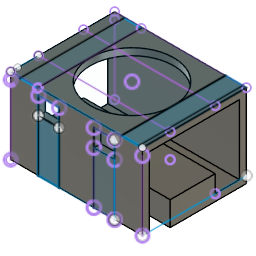
Movement Sensor (Autodesk Fusion 360 design; units mm, degrees)
part number: 2026-08-05-21-35-21-258
Autodesk Fusion 360 part; units mm, degrees
sketch "Sketch1" plane through (0, 0, 0) normal (0, 0, 1) x (1, 0, 0)
  line L0 (0, 0) -> (38, 0)
  line L1 (38, 0) -> (38, 30)
  line L2 (38, 30) -> (0, 30)
  line L3 (0, 30) -> (0, 0)
  line L4 (3, 3) -> (35, 3)
  line L5 (35, 3) -> (35, 27)
  line L6 (35, 27) -> (3, 27)
  line L7 (3, 27) -> (3, 3)
  line L8 (8, 27) -> (32, 27)
  line L9 (32, 27) -> (32, 3)
  line L10 (32, 3) -> (8, 3)
  line L11 (8, 3) -> (8, 27)
  circle A0 centre (20, 15) radius 12
  dimension "d1" = 38
  dimension "d2" = 30
  dimension "d3" = 32
  dimension "d4" = 24
  dimension "d5" = 3
  dimension "d6" = 3
  dimension "d7" = 24
  dimension "d8" = 24
  dimension "d9" = 5
  dimension "d11" = 3
  dimension "d12" = 24
  dimension "d13" = 12
  dimension "d14" = 16.9706
  constraint horizontal L0
  constraint vertical L1
  constraint horizontal L2
  constraint vertical L3
  constraint coincident L0.start L3.end
  constraint horizontal L4
  constraint vertical L5
  constraint horizontal L6
  constraint vertical L7
  constraint horizontal L8
  constraint vertical L9
  constraint horizontal L10
  constraint vertical L11
  measures "d1" distance of L0.start L0.end
  measures "d2" distance of L0.start L2.end
  measures "d3" distance of L4.start L4.end
  measures "d4" distance of L4.start L6.end
  measures "d5" distance of L3 L7
  measures "d6" distance of L2 L6
  measures "d7" distance of L8.start L8.end
  measures "d8" distance of L8.start L10.end
  measures "d9" distance of L7 L11
  measures "d11" distance of L2 L8
  measures "d12" diameter of A0
  measures "d13" distance of L9 A0.centre
  measures "d14" distance of L10.end A0.centre
sketch "Sketch2" plane through (0, 0, 0) normal (0, 1, 0) x (1, 0, 0)
  line L0 (0, 0) -> (38, 0)
  line L1 (38, 0) -> (38, 20)
  line L2 (38, 20) -> (0, 20)
  line L3 (0, 20) -> (0, 0)
  dimension "d15" = 38
  dimension "d16" = 20
  constraint horizontal L0
  constraint vertical L1
  constraint horizontal L2
  constraint vertical L3
  constraint coincident L0.start L3.end
  measures "d15" distance of L0.start L0.end
  measures "d16" distance of L0.start L2.end
sketch "Sketch3" plane through (0, 0, 0) normal (0, 1, 0) x (1, 0, 0)
  line L0 (8, 0) -> (14, 0)
  line L1 (14, 0) -> (14, 20)
  line L2 (14, 20) -> (8, 20)
  line L3 (8, 20) -> (8, 0)
  line L4 (0, 20) -> (0, 0)
  line L5 (24, 0) -> (30, 0)
  line L6 (30, 0) -> (30, 20)
  line L7 (30, 20) -> (24, 20)
  line L8 (24, 20) -> (24, 0)
  dimension "d17" = 6
  dimension "d18" = 20
  dimension "d19" = 8
  dimension "d21" = 6
  dimension "d22" = 20
  dimension "d23" = 10
  constraint horizontal L0
  constraint vertical L1
  constraint horizontal L2
  constraint vertical L3
  constraint horizontal L5
  constraint vertical L6
  constraint horizontal L7
  constraint vertical L8
  measures "d17" distance of L0.start L0.end
  measures "d18" distance of L0.start L2.end
  measures "d19" distance of L3 L4
  measures "d21" distance of L5.start L5.end
  measures "d22" distance of L5.start L7.end
  measures "d23" distance of L1 L8
sketch "Sketch4" plane through (0, 0, 0) normal (0, 1, 0) x (1, 0, 0)
sketch "Sketch5" plane through (0, 0, 0) normal (0, 1, 0) x (1, 0, 0)
sketch "Sketch6" plane through (0, 0, 0) normal (0, 1, 0) x (1, 0, 0)
  line L0 (8, 0) -> (14, 0)
  line L1 (14, 0) -> (14, 5)
  line L2 (14, 5) -> (8, 5)
  line L3 (8, 5) -> (8, 0)
  line L4 (38, 0) -> (38, 20)
  line L5 (14, 20) -> (8, 20)
  line L6 (14, 0) -> (14, 20)
  line L7 (24, 0) -> (30, 0)
  line L8 (30, 0) -> (30, 5)
  line L9 (30, 5) -> (24, 5)
  line L10 (24, 5) -> (24, 0)
  line L11 (38, 20) -> (0, 20)
  line L12 (0, 20) -> (0, 0)
  line L13 (30, 20) -> (24, 20)
  dimension "d24" = 5
  dimension "d25" = 24
  dimension "d26" = 15
  dimension "d27" = 6
  dimension "d28" = 15
  dimension "d29" = 14
  dimension "d30" = 30
  dimension "d31" = 20
  constraint horizontal L0
  constraint vertical L1
  constraint horizontal L2
  constraint vertical L3
  constraint horizontal L7
  constraint vertical L8
  constraint horizontal L9
  constraint vertical L10
  measures "d24" distance of L0.start L2.end
  measures "d25" distance of L1 L4
  measures "d26" distance of L2 L5
  measures "d27" distance of L3 L6
  measures "d28" distance of L9 L11
  measures "d29" distance of L4 L10
  measures "d30" distance of L8 L12
  measures "d31" distance of L7 L13
sketch "Sketch7" plane through (0, 0, 0) normal (1, 0, 0) x (0, 1, 0)
  line L0 (0, 0) -> (30, 0)
  line L1 (30, 0) -> (30, -20)
  line L2 (30, -20) -> (0, -20)
  line L3 (0, -20) -> (0, 0)
  line L4 (0, 0) -> (0, -20)
  line L5 (0, 0) -> (30, 0)
  dimension "d32" = 30
  dimension "d33" = 20
  constraint horizontal L0
  constraint vertical L1
  constraint horizontal L2
  constraint vertical L3
  constraint coincident L0.start L3.end
  measures "d32" distance of L1 L4
  measures "d33" distance of L2 L5
sketch "Sketch8" plane through (0, 0, 0) normal (0, 1, 0) x (1, 0, 0)
  line L0 (0, 20, 30) -> (38, 20, 30)
  line L1 (38, 20, 30) -> (38, 0, 30)
  line L2 (38, 0, 30) -> (0, 0, 30)
  line L3 (0, 0, 30) -> (0, 20, 30)
  dimension "d34" = 38
  dimension "d35" = 20
sketch "Sketch9" plane through (0, 0, 0) normal (1, 0, 0) x (0, 1, 0)
sketch "Sketch10" plane through (0, 30, 0) normal (0, 1, 0) x (-1, 0, 0)
sketch "Sketch11" plane through (0, 0, 0) normal (1, 0, 0) x (0, 1, 0)
  line L0 (0, -20, 38) -> (30, -20, 38)
sketch "Sketch12" plane through (0, 0, 0) normal (0, 0, 1) x (1, 0, 0)
sketch "Sketch13" plane through (0, 0, 0) normal (0, 0, 1) x (1, 0, 0)
sketch "Sketch14" plane through (0, 0, 0) normal (1, 0, 0) x (0, 1, 0)
  line L0 (8, -5) -> (21, -5)
  line L1 (21, -5) -> (21, -20)
  line L2 (21, -20) -> (8, -20)
  line L3 (8, -20) -> (8, -5)
  line L4 (30, -20) -> (30, 0)
  line L5 (0, 0) -> (30, 0)
  line L6 (0, 0) -> (0, -20)
  dimension "d36" = 15
  dimension "d37" = 9
  dimension "d38" = 5
  dimension "d39" = 8
  constraint horizontal L0
  constraint vertical L1
  constraint horizontal L2
  constraint vertical L3
  measures "d36" distance of L0.start L2.end
  measures "d37" distance of L1 L4
  measures "d38" distance of L0 L5
  measures "d39" distance of L3 L6
sketch "Sketch15" plane through (0, 0, 0) normal (1, 0, 0) x (0, 1, 0)
sketch "Sketch16" plane through (0, 0, 0) normal (0, 0, 1) x (1, 0, 0)
sketch "Sketch17" plane through (0, 0, 0) normal (1, 0, 0) x (0, 1, 0)
  line L0 (30, 0) -> (30, -20)
  line L1 (30, -20) -> (30, 0)
sketch "Sketch18" plane through (0, 0, 0) normal (1, 0, 0) x (0, 1, 0)
sketch "Sketch19" plane through (0, 30, 0) normal (0, 1, 0) x (1, 0, 0)
sketch "Sketch20" plane through (0, 0, 0) normal (1, 0, 0) x (0, 1, 0)
extrude "Extrude1" add sketch "Sketch1" along normal blind 2 contours L0 L1 L2 L3 | L4 L6 L7 L11 | L4 L10 L11 A0 | L4 L9 L10 A0 | L6 L8 L11 A0 | L4 L5 L6 L9 | L6 L8 L9 A0 makes body 1
extrude "Extrude2" add sketch "Sketch2" along normal blind 30 bodies 1
extrude "Extrude3" cut sketch "Sketch6" along normal blind 30 bodies 1
sketch "Sketch21" plane through (0, 0, 0) normal (0, -1, 0) x (1, 0, 0)
  line L0 (30, -5) -> (24, -5)
  line L1 (24, -5) -> (24, 0)
  line L2 (24, 0) -> (30, 0)
  line L3 (30, 0) -> (30, -5)
  line L4 (8, 0) -> (14, 0)
  line L5 (14, 0) -> (14, -5)
  line L6 (14, -5) -> (8, -5)
  line L7 (8, -5) -> (8, 0)
  line L8 (38, -20) -> (38, 2)
  line L9 (38, 2) -> (0, 2)
  line L10 (0, 2) -> (0, -20)
  line L11 (0, -20) -> (38, -20)
  line L12 (0, 0) -> (8, 0)
  line L13 (14, 0) -> (24, 0)
  line L14 (30, 0) -> (38, 0)
  constraint coincident L12.start origin
  constraint coincident L4.start L7.end
  constraint coincident L4.end L5.start
  constraint coincident L1.end L2.start
  constraint coincident L2.end L3.start
  constraint coincident L8 L14.end
  constraint perpendicular L8 L14
sketch "Sketch22" plane through (0, 0, 0) normal (0, -1, 0) x (1, 0, 0)
  line L0 (8, -5) -> (8, -20)
  line L1 (8, -20) -> (14, -20)
  line L2 (14, -20) -> (14, -5)
  line L3 (14, -20) -> (24, -20)
  line L4 (24, -20) -> (24, -5)
  line L5 (24, -5) -> (30, -5)
  line L6 (30, -5) -> (30, -20)
  dimension "d48" = 90
  dimension "d49" = 6
  constraint vertical L0
  constraint perpendicular L0 L1
  constraint perpendicular L1 L2
  constraint perpendicular L2 L3
  constraint perpendicular L1 L4
  constraint perpendicular L1 L6
  measures "d48" angle of L4 L5
  measures "d49" distance of L4.end L5.end
sketch "Sketch23" plane through (0, 0, 0) normal (0, -1, 0) x (1, 0, 0)
  line L0 (8, -5) -> (14, -5)
  line L1 (14, -5) -> (14, -20)
  line L2 (14, -20) -> (8, -20)
  line L3 (8, -20) -> (8, -5)
  line L4 (0, -20) -> (0, 0)
  line L5 (8, 0) -> (14, 0)
  line L6 (30, -20) -> (24, -20)
  line L7 (24, 0) -> (30, 0)
  line L8 (30, -5) -> (30, -20)
  line L9 (38, -20) -> (38, 0)
  line L10 (24, -20) -> (24, -5)
  dimension "d50" = 8
  dimension "d51" = 6
  dimension "d52" = 15
  dimension "d53" = 5
  dimension "d54" = 20
  dimension "d55" = 8
  dimension "d56" = 14
  constraint horizontal L0
  constraint vertical L1
  constraint horizontal L2
  constraint vertical L3
  measures "d50" distance of L3 L4
  measures "d51" distance of L1 L3
  measures "d52" distance of L0 L2
  measures "d53" distance of L0 L5
  measures "d54" distance of L6 L7
  measures "d55" distance of L8 L9
  measures "d56" distance of L9 L10
sketch "Sketch24" plane through (0, 0, 0) normal (0, -1, 0) x (1, 0, 0)
  line L0 (30, 0) -> (30, -20)
  constraint vertical L0
sketch "Sketch25" plane through (0, 0, 0) normal (0, 1, 0) x (1, 0, 0)
  line L0 (13.8134, -0.1132) -> (7.8134, -0.1132)
  line L1 (7.8134, -0.1132) -> (7.8134, 19.8868)
  line L2 (7.8134, 19.8868) -> (13.8134, 19.8868)
  line L3 (13.8134, 19.8868) -> (13.8134, -0.1132)
  dimension "d57" = 6
  dimension "d58" = 20
  constraint horizontal L0
  constraint vertical L1
  constraint horizontal L2
  constraint vertical L3
  measures "d57" distance of L0.start L0.end
  measures "d58" distance of L0.start L2.end
extrude "Extrude4" cut sketch "Sketch7" along normal blind 38 bodies 1
extrude "Extrude5" add sketch "Sketch14" along normal blind 38 separate body makes body 2
sketch "Sketch26" plane through (0, 0, 2) normal (0, 0, 1) x (-1, 0, 0)
  circle A0 centre (-20, -15) radius 12
  line L0 (0, -30) -> (0, 0)
  line L1 (0, 0) -> (-38, 0)
  line L2 (-38, 0) -> (-38, -30)
  line L3 (-38, -30) -> (0, -30)
  line L4 (0, -8) -> (-38, -8)
  line L5 (0, 0) -> (-8, 0)
  line L6 (0, -21) -> (-38, -21)
  line L7 (-38, -30) -> (0, -30)
  dimension "d63" = 8
  dimension "d64" = 38
  dimension "d65" = 38
  dimension "d66" = 9
  measures "d63" distance of L4 L5
  measures "d64" distance of L6.start L6.end
  measures "d65" distance of L2.end L0.start
  measures "d66" distance of L6 L7
extrude "Extrude6" add 1 faces at (12.6667, 16.6667, -20) along direction (0, 0, -1) blind 2 on bodies 2 bodies 2
sketch "Sketch27" plane through (0, 0, 2) normal (0, 0, 1) x (-1, 0, 0)
  line L0 (-32, -30.0218) -> (-37, -30.0218)
  line L1 (-37, -30.0218) -> (-37, -0.0218)
  line L2 (-37, -0.0218) -> (-32, -0.0218)
  line L3 (-32, -0.0218) -> (-32, -30.0218)
  line L4 (-3, -29.6627) -> (-8, -29.6627)
  line L5 (-8, -29.6627) -> (-8, 0.3373)
  line L6 (-8, 0.3373) -> (-3, 0.3373)
  line L7 (-3, 0.3373) -> (-3, -29.6627)
  point P0 (-20, -15)
  dimension "d69" = 5
  dimension "d70" = 30
  dimension "d71" = 12
  dimension "d72" = 5
  dimension "d73" = 30
  dimension "d74" = 12
  constraint horizontal L0
  constraint vertical L1
  constraint horizontal L2
  constraint vertical L3
  constraint horizontal L4
  constraint vertical L5
  constraint horizontal L6
  constraint vertical L7
  measures "d69" distance of L0.start L0.end
  measures "d70" distance of L0.start L2.end
  measures "d71" distance of L3 P0
  measures "d72" distance of L4.start L4.end
  measures "d73" distance of L4.start L6.end
  measures "d74" distance of P0 L5
extrude "Extrude7" add sketch "Sketch8" against normal blind 2 contours L0 L1 L2 L3 in plane through (0, 30, 0) normal (0, 1, 0) bodies 1
extrude "Extrude8" add sketch "Sketch21" against normal blind 2 contours L0 L1 L3 L5 L6 L7 L8 L10 L11 L12 L13 L14 bodies 1
sketch "Sketch28" plane through (0, 0, 2) normal (0, 0, 1) x (-1, 0, 0)
  line L0 (-32, -30) -> (-32, 0)
  line L1 (-32, 0) -> (-38, 0)
  line L2 (-38, 0) -> (-38, -30)
  line L3 (-38, -30) -> (-32, -30)
  line L4 (-8, -29.6627) -> (-8, 0.3373)
  line L5 (-38, 0) -> (0, 0)
  line L6 (0, -8) -> (0, -2)
  dimension "d79" = 6
  dimension "d80" = 24
  constraint vertical L0
  constraint perpendicular L0 L1
  constraint perpendicular L1 L2
  constraint horizontal L5
  constraint vertical L6
  measures "d79" distance of L0.end L1.end
  measures "d80" distance of L0 L4
sketch "Sketch29" plane through (0, 0, 0) normal (1, 0, 0) x (0, 1, 0)
  line L0 (30, -20) -> (21, -20)
  line L1 (21, -20) -> (21, -22)
  line L2 (21, -22) -> (30, -22)
  line L3 (30, -22) -> (30, -20)
  line L4 (8, -22) -> (8, -5)
  line L5 (-0.3373, 2) -> (29.6627, 2)
  dimension "d81" = 22
  dimension "d82" = 22
  dimension "d83" = 24
  dimension "d84" = 9
  constraint horizontal L0
  constraint vertical L1
  constraint horizontal L2
  constraint vertical L3
  measures "d81" distance of L2.end L4
  measures "d82" distance of L0 L5
  measures "d83" distance of L2 L5
  measures "d84" distance of L0.end L3
extrude "Extrude9" add sketch "Sketch29" along normal blind 38 bodies 1 2
sketch "Sketch30" plane through (38, 0, 0) normal (1, 0, 0) x (0, 1, 0)
  line L0 (2, 0) -> (28, 0)
  line L1 (28, 0) -> (28, -20)
  line L2 (28, -20) -> (21, -20)
  line L3 (8, -5) -> (8, -22)
  line L4 (8, -22) -> (30, -22)
  line L5 (30, -22) -> (30, 2)
  line L6 (30, 2) -> (0, 2)
  line L7 (0, 2) -> (0, -20)
  line L8 (0, -20) -> (2, -20)
  line L9 (2, -20) -> (2, 0)
sketch "Sketch31" plane through (38, 0, 0) normal (1, 0, 0) x (0, 1, 0)
  line L0 (2, 0) -> (28, 0)
  line L1 (28, 0) -> (28, -20)
  line L2 (28, -20) -> (21, -20)
  line L3 (8, -5) -> (8, -22)
  line L4 (8, -22) -> (30, -22)
  line L5 (30, -22) -> (30, 2)
  line L6 (30, 2) -> (0, 2)
  line L7 (0, 2) -> (0, -20)
  line L8 (0, -20) -> (2, -20)
  line L9 (2, -20) -> (2, 0)
sketch "Sketch33" plane through (38, 0, 0) normal (1, 0, 0) x (0, 1, 0)
  line L0 (8, -5) -> (20, -5)
  line L1 (20, -5) -> (20, -10)
  line L2 (20, -10) -> (8, -10)
  line L3 (8, -10) -> (8, -5)
  line L4 (8, -22) -> (30, -22)
  line L5 (2, -20) -> (2, 0)
  dimension "d89" = 12
  dimension "d90" = 5
  dimension "d91" = 6
  dimension "d92" = 12
  constraint horizontal L0
  constraint vertical L1
  constraint horizontal L2
  constraint vertical L3
  measures "d89" distance of L2 L4
  measures "d90" distance of L0 L2
  measures "d91" distance of L3 L5
  measures "d92" distance of L1 L3
extrude "Extrude10" cut sketch "Sketch33" against normal blind 38 bodies 1
extrude "Extrude11" cut 1 faces at (12.6667, 20.3333, -5) along direction (0, 0, -1) blind 5 on bodies 1 bodies 1
sketch "Sketch34" plane through (38, 0, 0) normal (1, 0, 0) x (0, 1, 0)
  line L0 (8, -10) -> (21, -10)
  line L1 (21, -10) -> (21, -15)
  line L2 (21, -15) -> (8, -15)
  line L3 (8, -15) -> (8, -10)
  line L4 (8, -22) -> (30, -22)
  dimension "d97" = 7
  dimension "d98" = 5
  constraint horizontal L0
  constraint vertical L1
  constraint horizontal L2
  constraint vertical L3
  measures "d97" distance of L2 L4
  measures "d98" distance of L0 L2
extrude "Extrude12" cut sketch "Sketch34" against normal blind 38 bodies 1
sketch "Sketch32" plane through (38, 0, 0) normal (1, 0, 0) x (0, 1, 0)
